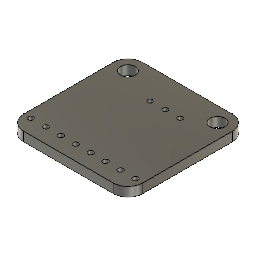
2809 LIS3DH (Autodesk Fusion 360 design; units mm, degrees)
Autodesk Fusion 360 part; units mm, degrees
sketch "Adafruit LIS3DH" plane through (0, 0, 0) normal (0, 0, 1) x (1, 0, 0)
  arc A0 (20.32, 17.78) -> (17.78, 20.32) centre (17.78, 17.78) ccw
  arc A1 (0, 2.54) -> (2.54, 0) centre (2.54, 2.54) ccw
  arc A2 (2.54, 20.32) -> (0, 17.78) centre (2.54, 17.78) ccw
  line L0 (17.78, 20.32) -> (2.54, 20.32)
  line L1 (2.54, 0) -> (17.78, 0)
  line L2 (0, 17.78) -> (0, 2.54)
  line L3 (20.32, 2.54) -> (20.32, 17.78)
  arc A3 (17.78, 0) -> (20.32, 2.54) centre (17.78, 2.54) ccw
  arc A4 (11.8745, 2.54) -> (10.9855, 2.54) centre (11.43, 2.54) ccw
  arc A5 (10.9855, 2.54) -> (11.8745, 2.54) centre (11.43, 2.54) ccw
  arc A6 (5.9055, 2.54) -> (6.7945, 2.54) centre (6.35, 2.54) ccw
  arc A7 (11.8491, 15.24) -> (11.0109, 15.24) centre (11.43, 15.24) ccw
  arc A8 (6.7945, 2.54) -> (5.9055, 2.54) centre (6.35, 2.54) ccw
  arc A9 (13.5509, 15.24) -> (14.3891, 15.24) centre (13.97, 15.24) ccw
  arc A10 (9.3091, 15.24) -> (8.4709, 15.24) centre (8.89, 15.24) ccw
  arc A11 (9.3345, 2.54) -> (8.4455, 2.54) centre (8.89, 2.54) ccw
  arc A12 (5.9055, 2.54) -> (6.7945, 2.54) centre (6.35, 2.54) ccw
  arc A13 (8.4709, 15.24) -> (9.3091, 15.24) centre (8.89, 15.24) ccw
  arc A14 (19.4945, 2.54) -> (18.6055, 2.54) centre (19.05, 2.54) ccw
  arc A15 (3.3655, 2.54) -> (4.2545, 2.54) centre (3.81, 2.54) ccw
  arc A16 (11.8491, 15.24) -> (11.0109, 15.24) centre (11.43, 15.24) ccw
  arc A17 (1.7145, 2.54) -> (0.8255, 2.54) centre (1.27, 2.54) ccw
  arc A18 (18.6055, 2.54) -> (19.4945, 2.54) centre (19.05, 2.54) ccw
  arc A19 (14.3891, 15.24) -> (13.5509, 15.24) centre (13.97, 15.24) ccw
  arc A20 (19.4945, 2.54) -> (18.6055, 2.54) centre (19.05, 2.54) ccw
  arc A21 (14.3891, 15.24) -> (13.5509, 15.24) centre (13.97, 15.24) ccw
  arc A22 (11.0109, 15.24) -> (11.8491, 15.24) centre (11.43, 15.24) ccw
  arc A23 (8.4455, 2.54) -> (9.3345, 2.54) centre (8.89, 2.54) ccw
  arc A24 (1.7145, 2.54) -> (0.8255, 2.54) centre (1.27, 2.54) ccw
  arc A25 (13.5255, 2.54) -> (14.4145, 2.54) centre (13.97, 2.54) ccw
  arc A26 (16.0655, 2.54) -> (16.9545, 2.54) centre (16.51, 2.54) ccw
  arc A27 (6.7945, 2.54) -> (5.9055, 2.54) centre (6.35, 2.54) ccw
  arc A28 (16.0655, 2.54) -> (16.9545, 2.54) centre (16.51, 2.54) ccw
  arc A29 (0.8255, 2.54) -> (1.7145, 2.54) centre (1.27, 2.54) ccw
  arc A30 (3.3655, 2.54) -> (4.2545, 2.54) centre (3.81, 2.54) ccw
  arc A31 (8.4455, 2.54) -> (9.3345, 2.54) centre (8.89, 2.54) ccw
  arc A32 (4.2545, 2.54) -> (3.3655, 2.54) centre (3.81, 2.54) ccw
  arc A33 (9.3091, 15.24) -> (8.4709, 15.24) centre (8.89, 15.24) ccw
  arc A34 (13.5255, 2.54) -> (14.4145, 2.54) centre (13.97, 2.54) ccw
  arc A35 (0.8255, 2.54) -> (1.7145, 2.54) centre (1.27, 2.54) ccw
  arc A36 (18.6055, 2.54) -> (19.4945, 2.54) centre (19.05, 2.54) ccw
  arc A37 (8.4709, 15.24) -> (9.3091, 15.24) centre (8.89, 15.24) ccw
  arc A38 (10.9855, 2.54) -> (11.8745, 2.54) centre (11.43, 2.54) ccw
  arc A39 (16.9545, 2.54) -> (16.0655, 2.54) centre (16.51, 2.54) ccw
  arc A40 (13.5509, 15.24) -> (14.3891, 15.24) centre (13.97, 15.24) ccw
  arc A41 (14.4145, 2.54) -> (13.5255, 2.54) centre (13.97, 2.54) ccw
  arc A42 (16.9545, 2.54) -> (16.0655, 2.54) centre (16.51, 2.54) ccw
  arc A43 (11.8745, 2.54) -> (10.9855, 2.54) centre (11.43, 2.54) ccw
  arc A44 (4.2545, 2.54) -> (3.3655, 2.54) centre (3.81, 2.54) ccw
  arc A45 (11.0109, 15.24) -> (11.8491, 15.24) centre (11.43, 15.24) ccw
  arc A46 (9.3345, 2.54) -> (8.4455, 2.54) centre (8.89, 2.54) ccw
  arc A47 (14.4145, 2.54) -> (13.5255, 2.54) centre (13.97, 2.54) ccw
  circle A48 centre (2.54, 17.78) radius 1.27
  circle A49 centre (17.78, 17.78) radius 1.27
  dimension "d3" = 2.54
  dimension "d4" = 2.54
  dimension "d5" = 17.78
  dimension "d6" = 2.54
  dimension "d7" = 17.78
  measures "d3" diameter of A48
  measures "d4" diameter of A49
  measures "d5" distance of L1 A2.centre
  measures "d6" distance of L2 A2.centre
  measures "d7" distance of L2 A0.centre
extrude "Extrude1" add sketch "Adafruit LIS3DH" along normal blind 1.6
